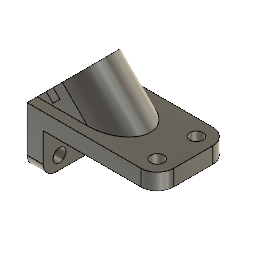
3D Plancha 9 (Autodesk Fusion 360 design; units mm, degrees)
Autodesk Fusion 360 part; units mm, degrees
sketch "Boceto1" plane through (0, 0, 0) normal (0, 0, 1) x (1, 0, 0)
  line L0 (0, 0) -> (0, 110)
  line L1 (0, 110) -> (200, 110)
  line L2 (200, 110) -> (200, 0)
  line L3 (200, 0) -> (0, 0)
  constraint coincident L0.start L3.end
  constraint vertical L0
  constraint perpendicular L0 L1
  constraint perpendicular L1 L2
  constraint perpendicular L2 L3
extrude "Extruir1" add sketch "Boceto1" along normal blind 90 makes body 1
fillet "Empalme1" radius 25 1 edges at (200, 0, 45) on bodies 1
fillet "Empalme2" radius 25 1 edges at (200, 110, 45) on bodies 1
sketch "Boceto2" plane through (0, 0, 90) normal (0, 0, 1) x (-1, 0, 0)
  arc A0 (-200, -85) -> (-175, -110) centre (-175, -85) ccw
  line L0 (-175, -110) -> (0, -110)
  line L1 (0, -110) -> (0, 0)
  line L2 (0, 0) -> (-175, 0)
  arc A1 (-175, 0) -> (-200, -25) centre (-175, -25) ccw
  line L3 (-200, -25) -> (-200, -85)
  circle A2 centre (-175, -25) radius 10
  circle A3 centre (-175, -85) radius 10
  dimension "d9" = 20
  dimension "d10" = 20
  constraint concentric A1 A2
  constraint concentric A0 A3
  measures "d9" diameter of A2
  measures "d10" diameter of A3
extrude "Extruir2" cut sketch "Boceto2" against normal blind 200 contours A2 | A3 bodies 1
fillet "Empalme3" radius 20 5 edges at (87.5, 110, 0) (192.6777, 102.6777, 0) (200, 55, 0) (192.6777, 7.3223, 0) (87.5, 0, 0) on bodies 1
sketch "Boceto3" plane through (0, 0, 0) normal (-1, 0, 0) x (0, -1, 0)
  arc A0 (-20, 0) -> (0, 20) centre (-20, 20) ccw
  line L0 (0, 20) -> (0, 90)
  line L1 (0, 90) -> (-110, 90)
  line L2 (-110, 90) -> (-110, 20)
  arc A1 (-110, 20) -> (-90, 0) centre (-90, 20) ccw
  line L3 (-90, 0) -> (-20, 0)
  circle A2 centre (-25, 20) radius 10
  circle A3 centre (-85, 20) radius 10
  dimension "d15" = 20
  dimension "d16" = 20
  measures "d15" diameter of A2
  measures "d16" diameter of A3
extrude "Extruir3" cut sketch "Boceto3" against normal blind 250 contours A2 | A3 bodies 1
move_body "Desplazar1" bodies 1 to x (1, 0, 0) y (0, 1, 0) z (0, 0, 1) at (110, 0, 0)
sketch "Boceto4" plane through (0, 0, 0) normal (1, 0, 0) x (0, 1, 0)
  line L0 (95.3327, 90.0002, 110) -> (15.3327, 90.0002, 110)
  line L1 (15.3327, 90.0002, 110) -> (15.3327, 157.1754, 177.1751)
  line L2 (15.3327, 157.1754, 177.1751) -> (95.3327, 157.1754, 177.1751)
  line L3 (95.3327, 157.1754, 177.1751) -> (95.3327, 90.0002, 110)
  point P0 (95.3327, 90.0002)
extrude "Extruir4" add sketch "Boceto4" along normal blind 100 contours L0 L1 L2 L3 in plane through (9.9999, 0, -9.9999) normal (0.707107, 0, -0.707107) bodies 1
fillet "Empalme4" radius 40 1 edges at (210.7628, 15.3327, 123.5877) on bodies 1
fillet "Empalme5" radius 40 1 edges at (210.7628, 95.3327, 123.5877) on bodies 1
sketch "Boceto5" plane through (9.9999, 0, -9.9999) normal (-0.707107, 0, 0.707107) x (0, -1, 0)
  arc A0 (-15.3327, 196.4215) -> (-95.3327, 196.4215) centre (-55.3327, 196.4215) ccw
  line L0 (-95.3327, 196.4215) -> (-95.3327, 141.4215)
  line L1 (-95.3327, 141.4215) -> (-15.3327, 141.4215)
  line L2 (-15.3327, 141.4215) -> (-15.3327, 196.4215)
  circle A1 centre (-55.3327, 196.4215) radius 15
  dimension "d28" = 30
  constraint concentric A0 A1
  measures "d28" diameter of A1
extrude "Extruir5" cut sketch "Boceto5" against normal blind 320 contours A1 bodies 1
sketch "Boceto6" plane through (9.9999, 0, -9.9999) normal (-0.707107, 0, 0.707107) x (0, -1, 0)
  circle A0 centre (-55.3327, 196.4215) radius 15
  arc A1 (-15.3327, 196.4215) -> (-95.3327, 196.4215) centre (-55.3327, 196.4215) ccw
  line L0 (-95.3327, 196.4215) -> (-95.3327, 141.4215)
  line L1 (-95.3327, 141.4215) -> (-15.3327, 141.4215)
  line L2 (-15.3327, 141.4215) -> (-15.3327, 196.4215)
  line L3 (-55.3327, 161.4215) -> (-15.3327, 161.4215)
  line L4 (-55.3327, 161.4215) -> (-95.3327, 161.4215)
  line L5 (-95.3327, 161.4215) -> (-95.3327, 176.4215)
  line L6 (-95.3327, 176.4215) -> (-15.3327, 176.4215)
  line L7 (-15.3327, 176.4215) -> (-15.3327, 161.4215)
  constraint coincident L2 L3.end
  constraint perpendicular L2 L3
  constraint coincident L0 L4.end
  constraint perpendicular L0 L4
  constraint perpendicular L4 L5
  constraint coincident L2 L6.end
  constraint perpendicular L2 L6
sketch "Boceto7" plane through (9.9999, 0, -9.9999) normal (-0.707107, 0, 0.707107) x (0, -1, 0)
extrude "Extruir6" cut sketch "Boceto6" against normal blind 15 contours L0 L2 L3 L4 L5 L6 L7 bodies 1
box "CajaPrimitiva1" add length 200 width 150 height 100 placed x (0, -1, 0) y (1, 0, 0) z (0, 0, 1) at (100, -60, 0) separate body makes body 2
move_body "Alinear1" bodies 2 to x (1, 0, 0) y (0, -1, 0) z (0, 0, -1) at (22.5, -60, 105)
move_body "Desplazar2" bodies 2 to x (1, 0, 0) y (0, 1, 0) z (0, 0, 1) at (-12.5, -30, -30)
move_body "Desplazar3" bodies 2 to x (1, 0, 0) y (0, 1, 0) z (0, 0, 1) at (25, 0, 0)
move_face "MoveFace1" by (0, 0, 10) 1 faces at (185, -30, 41.6667) on bodies 2
move_body "Desplazar4" bodies 2 to x (1, 0, 0) y (0, 1, 0) z (0, 0, 1) at (0, 0, 15)
move_body "Desplazar5" bodies 2 to x (1, 0, 0) y (0, 1, 0) z (0, 0, 1) at (0, 0, -25)
copy_body "CopiarPegarCuerpos1" bodies 2 makes body 3
move_body "Desplazar6" bodies 3 to x (1, 0, 0) y (0, 1, 0) z (0, 0, 1) at (150, 0, 0)
combine "Combinar1" operation cut target body 1 tool bodies 2 3
